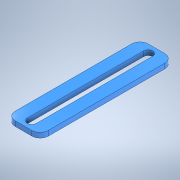
# Autodesk Inventor part: Carriage_Horizontal_Spacer
Saved by Autodesk Inventor 2021 (Build 250183000, 183)
## iProperties
Created: 2021-10-04
Part Number: Carriage_Horizontal_Spacer
Material: Generic
Document SubType Name: Modeling
Designer: Jorian Bruslind
Density: 1 g/cm^3
Appearance: Cyan
Author: Jorian Bruslind
Autodesk Inventor part; units mm, degrees
ref_plane "YZ Plane" through (0, 0, 0) normal (1, 0, 0) x (0, 1, 0)
ref_plane "XZ Plane" through (0, 0, 0) normal (0, 1, 0) x (-1, 0, 0)
ref_plane "XY Plane" through (0, 0, 0) normal (0, 0, 1) x (1, 0, 0)
sketch "Sketch1" plane through (0, 0, 0) normal (0, 1, 0) x (-1, 0, 0)
  line L0 (0, 0) -> (-20, 0)
  line L1 (-20, 0) -> (-20, -80)
  line L2 (-20, -80) -> (0, -80)
  line L3 (0, -80) -> (0, 0)
  line L4 (-10, 0) -> (-10, -5)
  line L5 (-10, -5) -> (-10, -75) construction
  line L6 (-12.75, -5) -> (-12.75, -75)
  line L7 (-7.25, -75) -> (-7.25, -5)
  arc A0 (-7.25, -5) -> (-12.75, -5) centre (-10, -5) ccw
  arc A1 (-12.75, -75) -> (-7.25, -75) centre (-10, -75) ccw
  line L8 (-10, -5) -> (60, -5) construction
  point P0 (-10, -40)
  dimension "d0" = 20
  dimension "d1" = 80
  dimension "d2" = 5
  dimension "d3" = 70
  dimension "d4" = 90
  dimension "d5" = 5.5
  constraints: 20 end point, 4 point on circle, 4 tangent, 3 parallel, 2 centre point, 2 horizontal, 2 midpoint, 2 perpendicular, 2 vertical
  measures "d0" distance of L2.end L1.end
  measures "d1" distance of L1.end L0.end
  measures "d2" distance of L4.start L4.end
  measures "d3" distance of L4.end L5.end
  measures "d4" angle of L5 L8
  measures "d5" diameter of A1
extrude "Extrusion1" add sketch "Sketch1" along normal blind 3
fillet "Fillet1" radius 5 4 edges at (20, 1.5, 0) (0, 1.5, 0) (20, 1.5, -80) (0, 1.5, -80)
body "Solid1"
